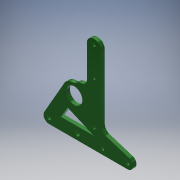
# Autodesk Inventor part: support plate 2
Saved by Autodesk Inventor 2017 SP1 (Build 210196100, 196)
## iProperties
Created: 2018-02-02
Part Number: support plate 2
Material: Generic
Document SubType Name: Modeling
Designer: Ben
Density: 1 g/cm^3
Appearance: Smooth - Dark Forest Green
Mass: 59.195 g
Surface Area: 246.284 cm^2
Volume: 59.195 cm^3
Author: Ben
Autodesk Inventor part; units mm, degrees
ref_plane "YZ Plane" through (0, 0, 0) normal (1, 0, 0) x (0, 1, 0)
ref_plane "XZ Plane" through (0, 0, 0) normal (0, 1, 0) x (-1, 0, 0)
ref_plane "XY Plane" through (0, 0, 0) normal (0, 0, 1) x (1, 0, 0)
sketch "0" plane through (0, 0, 0) normal (0, 0, 1) x (1, 0, 0)
  line L0 (0, -12.7) -> (-58.5803, -12.7)
  line L1 (-58.5803, -12.7) -> (-46.9681, 7.5534)
  line L2 (-46.9681, 7.5534) -> (0, -12.7)
  line L3 (12.7, 9.525) -> (12.7, 123.825)
  arc A0 (12.7, 123.825) -> (-12.7, 123.825) centre (0, 123.825) ccw
  line L4 (-12.7, 123.825) -> (-12.7, 66.675)
  arc A1 (-22.225, 57.15) -> (-12.7, 66.675) centre (-22.225, 66.675) ccw
  arc A2 (-22.225, 57.15) -> (-30.1625, 53.975) centre (-22.225, 45.6406) ccw
  arc A3 (-38.1, 50.8) -> (-30.1625, 53.975) centre (-38.1, 62.3094) ccw
  arc A4 (-38.1, 50.8) -> (-52.6123, 42.3922) centre (-38.1, 34.0717) ccw
  line L5 (-52.6123, 42.3922) -> (-88.4002, -20.0273)
  arc A5 (-88.4002, -20.0273) -> (-80.137, -34.29) centre (-80.137, -24.765) ccw
  line L6 (-80.137, -34.29) -> (59.563, -34.29)
  arc A6 (59.563, -34.29) -> (62.4705, -15.6946) centre (59.563, -24.765) ccw
  line L7 (62.4705, -15.6946) -> (21.5233, -2.5688)
  arc A7 (12.7, 9.525) -> (21.5233, -2.5688) centre (25.4, 9.525) ccw
  circle A8 centre (0, 0) radius 2.667
  circle A9 centre (0, 76.2) radius 2.667
  circle A10 centre (0, 127) radius 2.667
  circle A11 centre (-34.925, 31.75) radius 14.2875
  line L8 (0, 127) -> (0, 0) construction
  line L9 (-84.1991, -12.7) -> (53.1285, -12.7) construction
  line L10 (-22.225, 57.15) -> (0, 57.15) construction
  line L11 (-38.1, 50.8) -> (0, 50.8) construction
  line L12 (-52.8286, 42.0149) -> (-47.3198, 38.8565) construction
  line L13 (-45.6113, 6.9684) -> (-40.5824, 18.6303) construction
  circle A12 centre (-80.137, -24.765) radius 3.3528 projected
  circle A13 centre (-29.9986, -24.257) radius 4.064 projected
  circle A14 centre (14.7822, -24.511) radius 3.3528 projected
  circle A15 centre (59.563, -24.765) radius 3.3528 projected
  line L14 (-34.925, 50.8) -> (-34.925, 46.0375) construction
  dimension "d0" = 5.334
  dimension "d1" = 76.2
  dimension "d2" = 127
  dimension "d3" = 12.7
  dimension "d4" = 3.175
  dimension "d6" = 28.575
  dimension "d8" = 12.7
  dimension "d9" = 12.7
  dimension "d12" = 57.15
  dimension "d13" = 6.35
  dimension "d14" = 34.925
  dimension "d15" = 44.45
  dimension "d16" = 6.35
  dimension "d25" = 9.525
  dimension "d26" = 12.7
  dimension "d27" = 22.225
  dimension "d28" = 22.225
  dimension "d29" = 12.7
  dimension "d35" = 9.525
  dimension "d36" = 25.4
  dimension "d37" = 4.7625
  constraints: 30 end point, 19 point on circle, 14 tangent, 13 point on line, 12 centre point, 4 equal radius, 4 perpendicular, 3 vertical, 2 coincident, 1 collinear, 1 horizontal, 1 parallel
  measures "d0" diameter of A8
  measures "d1" distance of L8.end A9.centre
  measures "d2" distance of L8.start L8.end
  measures "d3" radius of A0
  measures "d4" distance of L8.start A0.centre
  measures "d6" diameter of A11
  measures "d8" distance from line of L8.end L9
  measures "d9" distance between parallel lines of L8 L3
  measures "d12" distance from line of L8.end L10
  measures "d13" distance between parallel lines of L11 L10
  measures "d14" distance from line of L8 A11.centre
  measures "d15" distance from line of L9 A11.centre
  measures "d16" distance of L12.start L12.end
  measures "d25" radius of A6
  measures "d26" radius of A7
  measures "d27" distance from line of L9 L3.start
  measures "d28" distance between parallel lines of L5 L1
  measures "d29" distance of L13.start L13.end
  measures "d35" distance from line of L4 L10.start
  measures "d36" distance from line of L4 L11.start
  measures "d37" distance of L14.start L14.end
extrude "Extrusion1" add sketch "0" along normal blind 6.35
chamfer "Chamfer1" distance 2.3813 angle 45 3 edges at (-2.667, 127, 0) (-2.667, 76.2, 0) (-2.667, 0, 0)
body "Solid1"
